Autodesk Inventor part; units mm, degrees
(part 2 of 2)
ref_plane "to_Plug_1_2_XY" through (-255, 0, -80) normal (0, 1, 0) x (1, 0, 0)
ref_plane "to_Plug_1_2_YZ" through (-255, 0, -80) normal (1, 0, 0) x (0, 0, -1)
ref_plane "to_Plug_1_2_ZX" through (-255, 0, -80) normal (0, 0, -1) x (0, 1, 0)
ref_plane "to_Plug_1_3_XY" through (255, 0, 107.5) normal (0, 1, 0) x (1, 0, 0)
ref_plane "to_Plug_1_3_YZ" through (255, 0, 107.5) normal (1, 0, 0) x (0, 0, -1)
ref_plane "to_Plug_1_3_ZX" through (255, 0, 107.5) normal (0, 0, -1) x (0, 1, 0)
ref_plane "to_Plug_1_4_XY" through (-255, 0, 107.5) normal (0, 1, 0) x (1, 0, 0)
ref_plane "to_Plug_1_4_YZ" through (-255, 0, 107.5) normal (1, 0, 0) x (0, 0, -1)
ref_plane "to_Plug_1_4_ZX" through (-255, 0, 107.5) normal (0, 0, -1) x (0, 1, 0)
body "Solid1"
